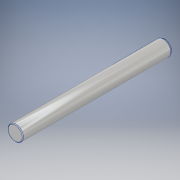
# Autodesk Inventor part: NEMA_14HM11-0404S_SHAFT
Saved by Autodesk Inventor 2019.4 (Build 234330000, 330)
## iProperties
Created: 2019-11-25
Part Number: NEMA_14HM11-0404S_SHAFT
Material: Générique
Document SubType Name: Modeling
Designer: thoma
Density: 1 g/cm^3
Appearance: Aluminium - Plat
Author: thoma
Autodesk Inventor part; units mm, degrees
ref_plane "YZ Plane" through (0, 0, 0) normal (1, 0, 0) x (0, 1, 0)
ref_plane "XZ Plane" through (0, 0, 0) normal (0, 1, 0) x (-1, 0, 0)
ref_plane "XY Plane" through (0, 0, 0) normal (0, 0, 1) x (1, 0, 0)
sketch "Esquisse1" plane through (0, 0, 0) normal (0, 0, 1) x (1, 0, 0)
  circle A0 centre (0, 0) radius 2.5
  dimension "d0" = 5
  constraints: 1 centre point, 1 coincident
  measures "d0" diameter of A0
extrude "Extrusion1" add sketch "Esquisse1" against normal blind 49
chamfer "Chanfrein1" distance 0.2 angle 45 1 edges at (-2.5, 0, 0)
chamfer "Chanfrein2" distance 0.3 angle 60 1 edges at (-2.5, 0, -49) measured on face at (-2, 0, -49)
sketch "Esquisse2" plane through (0, 0, -49) normal (0, 0, -1) x (-1, 0, 0)
  circle A0 centre (0, 0) radius 2.5 construction
  line L0 (-2.5, 0) -> (2, 0) construction
  line L1 (2, 0) -> (2, 1.5)
  line L2 (2, 0) -> (2, -1.5)
  arc A1 (2, -1.5) -> (2, 1.5) centre (0, 0) ccw
  dimension "d9" = 4.5
  constraints: 6 end point, 2 point on circle, 1 centre point, 1 coincident, 1 horizontal, 1 horizontal alignment, 1 point on line, 1 vertical, 1 other
  measures "d9" distance of L0.start L0.end
extrude "Extrusion2" cut sketch "Esquisse2" against normal blind 15
fillet "Congé1" radius 0.1 3 edges at (-2, 0, -49) (-2, 1.1989, -48.7717) (-2, -1.1989, -48.7717)
